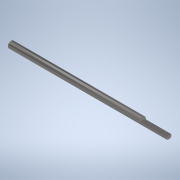
# Autodesk Inventor part: rat_headbarStraight
Saved by Autodesk Inventor 2021 (Build 250183000, 183)
## iProperties
Created: 2016-02-18
Part Number: rat_headbarStraight
Material: Stainless Steel
Document SubType Name: Modeling
Designer: Ariel
Density: 8 g/cm^3
Appearance: Semi-Polished
Author: Ariel
Autodesk Inventor part; units mm, degrees
ref_plane "YZ Plane" through (0, 0, 0) normal (1, 0, 0) x (0, 1, 0)
ref_plane "XZ Plane" through (0, 0, 0) normal (0, 1, 0) x (-1, 0, 0)
ref_plane "XY Plane" through (0, 0, 0) normal (0, 0, 1) x (1, 0, 0)
sketch "Sketch1" plane through (0, 0, 0) normal (1, 0, 0) x (0, 1, 0)
  circle A0 centre (0, 0) radius 6.35
  dimension "d61" = 12.7
  constraints: 1 centre point, 1 coincident
  measures "d61" diameter of A0
extrude "Extrusion1" add sketch "Sketch1" against normal blind 304.8
sketch "Sketch2" plane through (0, 0, 0) normal (1, 0, 0) x (0, 0, -1)
  arc A0 (6.35, 0) -> (-6.35, 0) centre (0, 0) ccw
  circle A1 centre (0, 0) radius 6.35 projected
  line L0 (-6.35, 0) -> (6.35, 0)
  constraints: 4 point on circle, 3 end point, 1 centre point, 1 coincident, 1 horizontal, 1 midpoint
extrude "Extrusion2" cut sketch "Sketch2" against normal blind 50.8 contours L0 A0
sketch "Sketch3" plane through (0, 0, 6.35) normal (0, 1, 0) x (1, 0, 0)
  circle A0 centre (-12.468, 6.35) radius 1.5875
  circle A1 centre (-4.5305, 6.35) radius 1.5875
  line L0 (0, 6.35) -> (-2.943, 6.35)
  line L1 (0, 12.7) -> (0, 0) projected
  line L2 (-2.943, 6.35) -> (-12.468, 6.35) construction
  dimension "d50" = 3.175
  dimension "d48" = 7.9375
  dimension "d49" = 3.175
  dimension "d60" = 2.943
  constraints: 5 end point, 2 horizontal, 1 centre point, 1 coincident, 1 horizontal alignment, 1 perpendicular, 2 other
  measures "d48" distance of point (-4.53, 6.35) L2.end
  measures "d49" diameter of A0
  measures "d60" distance of L0.start L0.end
sketch "Sketch5" plane through (0, 0, 6.35) normal (0, 1, 0) x (1, 0, 0)
  line L0 (0, 6.35) -> (0, 11.176)
  line L1 (0, 12.7) -> (0, 0) projected
  line L2 (0, 11.176) -> (-50.8, 11.176)
  line L3 (-50.8, 12.7) -> (-50.8, 0) projected
  line L4 (0, 6.35) -> (0, 1.524)
  line L5 (0, 1.524) -> (-50.8, 1.524)
  line L6 (-50.8, 1.524) -> (-50.8, -4.826)
  line L7 (-50.8, -4.826) -> (10.9985, -4.826)
  line L8 (10.9985, -4.826) -> (0, 1.524)
  line L9 (-50.8, 11.176) -> (-50.8, 17.526)
  line L10 (-50.8, 17.526) -> (10.9985, 17.526)
  line L11 (0, 11.176) -> (10.9985, 17.526)
  line L12 (-50.8, 12.7) -> (0, 12.7) projected
  dimension "d20" = 4.826
  dimension "d21" = 4.826
  dimension "d62" = 4.826
  constraints: 20 end point, 4 equal length, 4 point on line, 2 horizontal, 2 vertical, 1 perpendicular
  measures "d20" distance of L0.start L0.end
  measures "d21" distance of L0.start L4.end
  measures "d62" distance between parallel lines of L12 L10
extrude "Extrusion3" cut sketch "Sketch5" against normal blind 25.4 contours L2 L3 L12 L1 | L1 L12 L9 L10 L11 | L8 L7 L6 L3 L5
hole "Hole3" at (-12.468, 0, 0) at (-4.5305, 0, 0) direction (0, -1, 0) diameter 2.4867 end through all thread size "5-40 UNC" class "2B" standard "ANSI Unified Screw Threads"
equation "\"d62\" = d20"
body "Solid1"
